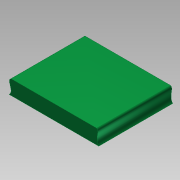
# Autodesk Inventor part: DO-214AB (SMC) плата
Saved by Autodesk Inventor 2011 (Build 150239000, 239)
## iProperties
Created: 2011-01-13
Part Number: DO-214AB (SMC) плата
Document SubType Name: Modeling
Designer: abbath
Density: 1 g/cm^3
Author: abbath
Autodesk Inventor part; units mm, degrees
ref_plane "YZ Plane" through (0, 0, 0) normal (1, 0, 0) x (0, 1, 0)
ref_plane "XZ Plane" through (0, 0, 0) normal (0, 1, 0) x (-1, 0, 0)
ref_plane "XY Plane" through (0, 0, 0) normal (0, 0, 1) x (1, 0, 0)
sketch "Эскиз1" plane through (0, 0, 0) normal (0, 0, 1) x (1, 0, 0)
  line L0 (-2.3836, -3.6179) -> (7.4736, -3.6179)
  line L1 (7.4736, -3.6179) -> (7.4736, 3.9975)
  line L2 (7.4736, 3.9975) -> (-2.3836, 3.9975)
  line L3 (-2.3836, 3.9975) -> (-2.3836, -3.6179)
  point P0 (0, 0)
  constraints: 8 end point, 2 parallel, 1 horizontal, 1 perpendicular
extrude "Выдавливание1" add sketch "Эскиз1" along normal blind 1.5
sketch "Эскиз2" plane through (-2.3836, -3.6179, 0) normal (0, -1, 0) x (1, 0, 0)
  line L0 (9.8572, 1.5) -> (0, 1.5) projected
  line L1 (0, 0) -> (0, 1.5) projected
  line L2 (0, 0) -> (9.8572, 0) projected
  line L3 (9.8572, 0) -> (9.8572, 1.5) projected
  spline S0 degree 3 poles (9.5515, 0) (9.1059, 0.5057) (9.6806, 1.3196) (9.3312, 1.5) knots 0 0 0 0 1 1 1 1
  spline S1 degree 3 poles (0.3074, 0) (0.9015, 0.4878) (-0.001, 1.222) (0.5194, 1.5) knots 0 0 0 0 1 1 1 1
  point P0 (2.3836, 0)
  point P1 (9.3821, 0.6943)
  point P2 (9.4499, 1.2761)
  point P3 (0.5013, 0.6008)
  point P4 (0.3525, 1.1779)
  constraints: 4 point on line, 8 other
extrude "Выдавливание2" cut sketch "Эскиз2" against normal through all contours L3 L2 S0 L0 | S1 L2 L1 L0
